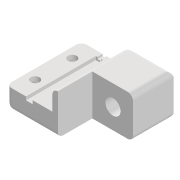
# Autodesk Inventor part: NadelhalterSchraub
Saved by Autodesk Inventor 2022 (Build 260153000, 153)
## iProperties
Created: 2021-05-31
Part Number: NadelhalterSchraub
Material: Generisch
Document SubType Name: Modeling
Designer: Sven
Density: 1 g/cm^3
Appearance: Vorgabe
Author: Sven
Autodesk Inventor part; units mm, degrees
ref_plane "YZ Plane" through (0, 0, 0) normal (1, 0, 0) x (0, 1, 0)
ref_plane "XZ Plane" through (0, 0, 0) normal (0, 1, 0) x (-1, 0, 0)
ref_plane "Arbeitsebene1" through (0, 0, -12.7) normal (0, 0, -1) x (-1, 0, 0)
sketch "Skizze2" plane through (0, 0, -12.7) normal (0, 0, -1) x (-1, 0, 0)
  line L0 (-55.25, 0) -> (-55.25, -12.7) projected
  line L1 (0, -12.7) -> (-55.25, -12.7) projected
  line L2 (0, 0) -> (0, -12.7) projected
  line L3 (0, 0) -> (-55.25, 0) projected
  circle A0 centre (-47.625, -6.35) radius 2.75 projected
  circle A1 centre (-7.625, -6.35) radius 2.75 projected
  line L4 (0, 1.15) -> (-15, 1.15)
  line L5 (-15, 1.15) -> (-15, -13.85)
  line L6 (-15, -13.85) -> (0, -13.85)
  line L7 (0, -13.85) -> (0, 1.15)
  point P0 (-15, -6.35)
  dimension "d1" = 15
  dimension "d2" = 0
  dimension "d3" = 15
  constraints: 8 end point, 2 parallel, 1 horizontal, 1 horizontal alignment, 1 midpoint, 1 perpendicular
  measures "d1" distance of L4.end L5.end
  measures "d2" distance between parallel lines of L2 L7
  measures "d3" distance between parallel lines of L2 L5
extrude "Extrusion1" add sketch "Skizze2" along normal blind 15 contours L5 L4 L7 L3 | L3 L2 L1 L5 | L1 L7 L6 L5 | A1
sketch "Skizze3" plane through (0, -13.85, -12.7) normal (-1, 0, 0) x (0, 0, 1)
  line L0 (12.7, 1.15) -> (12.7, 13.85) projected
  line L1 (-15, 0) -> (-15, 15) projected
  line L2 (-15, 15) -> (12.7, 15)
  line L3 (12.7, 15) -> (12.7, 0)
  line L4 (12.7, 0) -> (-15, 0)
  line L5 (-15, 0) -> (-15, 15)
  line L6 (0, 0) -> (-15, 0) projected
  constraints: 8 end point, 2 collinear, 2 parallel, 1 horizontal, 1 perpendicular
extrude "Extrusion2" add sketch "Skizze3" along normal blind 2
sketch "Skizze4" plane through (-2, -13.85, -12.7) normal (-1, 0, 0) x (0, 0, 1)
  line L0 (0, 0) -> (12.7, 0) projected
  line L1 (-15, 15) -> (-15, 0) projected
  line L2 (12.7, 0) -> (-15, 0)
  line L3 (-15, 0) -> (-15, 7.5)
  line L4 (-15, 7.5) -> (12.7, 7.5)
  line L5 (12.7, 7.5) -> (12.7, 0)
  line L6 (12.7, 0) -> (12.7, 15) projected
  point P0 (12.7, 13.85)
  point P1 (12.7, 7.5)
  point P2 (-1.15, 7.5)
  constraints: 8 end point, 3 midpoint, 2 parallel, 1 horizontal, 1 horizontal alignment, 1 perpendicular
extrude "Extrusion3" add sketch "Skizze4" along normal blind 17
sketch "Skizze5" plane through (-2, -6.35, 0) normal (0, 1, 0) x (1, 0, 0)
  line L0 (0, 27.7) -> (-17, 27.7) projected
  line L1 (0, 0) -> (0, 27.7) projected
  line L2 (0, 0) -> (-17, 0) projected
  line L3 (-17, 0) -> (-17, 27.7) projected
  line L4 (-7.25, 0) -> (-9.75, 0)
  line L5 (-9.75, 0) -> (-9.75, 25.75)
  line L6 (-9.75, 25.75) -> (-7.25, 25.75)
  line L7 (-7.25, 25.75) -> (-7.25, 0)
  point P0 (2, 0)
  point P1 (-8.5, 0)
  point P2 (-8.5, 0)
  dimension "d10" = 2.5
  dimension "d17" = 25.75
  constraints: 8 end point, 2 midpoint, 2 parallel, 1 coincident, 1 horizontal, 1 perpendicular, 1 point on line
  measures "d10" distance of L5.end L6.end
  measures "d17" distance between parallel lines of L6 L2
extrude "Extrusion4" cut sketch "Skizze5" against normal blind 1.25 contours L2 L5 L6 L7
sketch "Skizze6" plane through (-2, -6.35, 0) normal (0, 1, 0) x (1, 0, 0)
  line L0 (-9.75, 25.75) -> (-7.25, 25.75) projected
  line L1 (-7.25, 25.75) -> (-7.25, 0) projected
  line L2 (-9.75, 0) -> (-9.75, 25.75) projected
  line L3 (0, 27.7) -> (-17, 27.7) projected
  line L4 (-9.75, 25.75) -> (-7.25, 25.75) projected
  line L5 (-7.8, 25.75) -> (-9.2, 25.75)
  line L6 (-9.2, 25.75) -> (-9.2, 27.7)
  line L7 (-9.2, 27.7) -> (-7.8, 27.7)
  line L8 (-7.8, 27.7) -> (-7.8, 25.75)
  point P0 (2, 0)
  point P1 (-8.5, 25.75)
  point P2 (-8.5, 25.75)
  point P3 (-7.8, 27.7)
  dimension "d14" = 1.4
  constraints: 8 end point, 2 midpoint, 2 parallel, 2 point on line, 1 coincident, 1 horizontal, 1 perpendicular
  measures "d14" distance between parallel lines of L6 L8
extrude "Extrusion5" cut sketch "Skizze6" against normal blind 0.7
sketch "Skizze7" plane through (-2, -6.35, 0) normal (0, 1, 0) x (1, 0, 0)
  circle A0 centre (-3.625, 7) radius 2
  circle A1 centre (-13.375, 7) radius 2
  circle A2 centre (-13.375, 20.7) radius 2
  circle A3 centre (-3.625, 20.7) radius 2
  line L0 (0, 0) -> (-7.25, 0) projected
  line L1 (-9.75, 0) -> (-17, 0) projected
  line L2 (-9.2, 27.7) -> (-17, 27.7) projected
  point P0 (2, 0)
  point P1 (-3.625, 0)
  point P2 (-13.375, 0)
  dimension "d18" = 4
  dimension "d19" = 4
  dimension "d20" = 4
  dimension "d21" = 4
  dimension "d22" = 7
  dimension "d23" = 7
  constraints: 4 centre point, 4 vertical alignment, 2 horizontal alignment, 2 midpoint
  measures "d18" diameter of A0
  measures "d19" diameter of A1
  measures "d20" diameter of A2
  measures "d21" diameter of A3
  measures "d22" distance from line of A0.centre L0
  measures "d23" distance from line of A2.centre L2
extrude "Extrusion6" cut sketch "Skizze7" against normal blind 10
sketch "Skizze9" plane through (0, 0, -27.7) normal (0, 0, -1) x (-1, 0, 0)
  circle A0 centre (-7.625, -6.35) radius 2.75 projected
  point P0 (0, 0)
  constraints: 1 coincident
hole "Bohrung1" at (7.625, -6.35, -27.7) direction (0, 0, 1) diameter 5.6 depth 15 counterbore diameter 9 counterbore depth 6
sketch "Skizze10" plane through (0, 1.15, -12.7) normal (0, 1, 0) x (1, 0, 0)
  line L0 (19, -16) -> (-4, -16)
  line L1 (-4, -16) -> (-4, 20)
  line L2 (-4, 20) -> (19, 20)
  line L3 (19, 20) -> (19, -16)
  point P0 (0, -12.7)
  constraints: 8 end point, 2 parallel, 1 horizontal, 1 perpendicular
extrude "Extrusion8" cut sketch "Skizze10" against normal blind 1.15
sketch "Skizze11" plane through (15, -13.85, -27.7) normal (0, -1, 0) x (1, 0, 0)
  line L0 (6, 49) -> (-39, 49)
  line L1 (-39, 49) -> (-39, -17)
  line L2 (-39, -17) -> (6, -17)
  line L3 (6, -17) -> (6, 49)
  point P0 (-15, 27.7)
  constraints: 8 end point, 2 parallel, 1 horizontal, 1 perpendicular
extrude "Extrusion9" cut sketch "Skizze11" against normal blind 1.15
fillet "Rundung2" radius 2 5 edges at (-19, -9.525, -27.7) (-19, -9.525, 0) (15, -6.35, -27.7) (15, 0, -20.2) (6.5, 0, -27.7)
equation "\"d19\" = d18"
equation "\"d20\" = d19"
equation "\"d21\" = d19"
equation "\"d23\" = d22"
